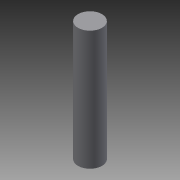
# Autodesk Inventor part: Biztositek15mm
Saved by Autodesk Inventor 2015 (Build 190159000, 159)
## iProperties
Created: 2014-10-20
Part Number: Biztositek15mm
Material: Generic
Document SubType Name: Modeling
Designer: laca
Density: 1 g/cm^3
Appearance: Default
Mass: 0.106029 g
Surface Area: 1.55509 cm^2
Volume: 0.106029 cm^3
Author: laca
Autodesk Inventor part; units mm, degrees
ref_plane "YZ Plane" through (0, 0, 0) normal (1, 0, 0) x (0, 1, 0)
ref_plane "XZ Plane" through (0, 0, 0) normal (0, 1, 0) x (-1, 0, 0)
ref_plane "XY Plane" through (0, 0, 0) normal (0, 0, 1) x (1, 0, 0)
sketch "Sketch1" plane through (0, 0, 0) normal (0, 1, 0) x (-1, 0, 0)
  circle A0 centre (-2.5419, -6.6374) radius 1.5
  point P0 (0, 0)
  dimension "d0" = 3
  dimension "d0" = 3
  constraints: 1 centre point
  measures "d0" diameter of A0
extrude "Extrusion1" add sketch "Sketch1" along normal blind 15
body "Solid1"
